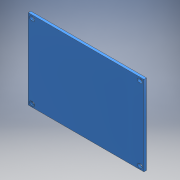
# Autodesk Inventor part: screen
Saved by Autodesk Inventor 2017 (Build 210142000, 142)
## iProperties
Part Number: screen
Material: Genérico
Document SubType Name: Modeling
Designer: Roberto
Density: 1 g/cm^3
Appearance: Valor por defecto
Author: Roberto
Autodesk Inventor part; units mm, degrees
ref_plane "YZ Plane" through (0, 0, 0) normal (1, 0, 0) x (0, 1, 0)
ref_plane "XZ Plane" through (0, 0, 0) normal (0, 1, 0) x (-1, 0, 0)
sketch "Boceto6" plane through (0, 0, 0) normal (0, 1, 0) x (-1, 0, 0)
  line L0 (0, 0) -> (8.94, 0)
  line L1 (8.94, 0) -> (8.94, -6.196)
  line L2 (8.94, -6.196) -> (0, -6.196)
  line L3 (0, -6.196) -> (0, 0)
  arc A0 (0.25, -0.1) -> (0.25, -0.4) centre (0.25, -0.25) ccw
  arc A1 (0.35, -0.4) -> (0.35, -0.1) centre (0.35, -0.25) ccw
  line L4 (0.25, -0.4) -> (0.35, -0.4)
  line L5 (0.25, -0.1) -> (0.35, -0.1)
  arc A2 (8.59, -0.1) -> (8.59, -0.4) centre (8.59, -0.25) ccw
  arc A3 (8.69, -0.4) -> (8.69, -0.1) centre (8.69, -0.25) ccw
  line L6 (8.59, -0.4) -> (8.69, -0.4)
  line L7 (8.59, -0.1) -> (8.69, -0.1)
  arc A4 (0.25, -5.796) -> (0.25, -6.096) centre (0.25, -5.946) ccw
  arc A5 (0.35, -6.096) -> (0.35, -5.796) centre (0.35, -5.946) ccw
  line L8 (0.25, -6.096) -> (0.35, -6.096)
  line L9 (0.25, -5.796) -> (0.35, -5.796)
  arc A6 (8.59, -5.796) -> (8.59, -6.096) centre (8.59, -5.946) ccw
  arc A7 (8.69, -6.096) -> (8.69, -5.796) centre (8.69, -5.946) ccw
  line L10 (8.59, -6.096) -> (8.69, -6.096)
  line L11 (8.59, -5.796) -> (8.69, -5.796)
  constraints: 24 end point, 16 point on circle, 8 centre point
extrude "Extrusión4" add sketch "Boceto6" along normal blind 0.6
sketch "Boceto7" plane through (0, 0.6, 0) normal (0, 1, 0) x (1, 0, 0)
  line L0 (-8.59, 5.796) -> (-8.69, 5.796) projected
  arc A0 (-8.69, 6.096) -> (-8.69, 5.796) centre (-8.69, 5.946) ccw projected
  line L1 (-8.69, 6.096) -> (-8.59, 6.096) projected
  arc A1 (-8.59, 5.796) -> (-8.59, 6.096) centre (-8.59, 5.946) ccw projected
  line L2 (-0.25, 5.796) -> (-0.35, 5.796) projected
  arc A2 (-0.35, 6.096) -> (-0.35, 5.796) centre (-0.35, 5.946) ccw projected
  line L3 (-0.35, 6.096) -> (-0.25, 6.096) projected
  arc A3 (-0.25, 5.796) -> (-0.25, 6.096) centre (-0.25, 5.946) ccw projected
  line L4 (-8.59, 0.1) -> (-8.69, 0.1) projected
  arc A4 (-8.69, 0.4) -> (-8.69, 0.1) centre (-8.69, 0.25) ccw projected
  line L5 (-8.69, 0.4) -> (-8.59, 0.4) projected
  arc A5 (-8.59, 0.1) -> (-8.59, 0.4) centre (-8.59, 0.25) ccw projected
  line L6 (-0.25, 0.1) -> (-0.35, 0.1) projected
  arc A6 (-0.35, 0.4) -> (-0.35, 0.1) centre (-0.35, 0.25) ccw projected
  line L7 (-0.35, 0.4) -> (-0.25, 0.4) projected
  arc A7 (-0.25, 0.1) -> (-0.25, 0.4) centre (-0.25, 0.25) ccw projected
  line L8 (-8.94, 0) -> (0, 0) projected
  line L9 (0, 0) -> (0, 6.196) projected
  line L10 (0, 6.196) -> (-8.94, 6.196) projected
  line L11 (-8.94, 6.196) -> (-8.94, 0) projected
  line L12 (-8.94, 6.196) -> (0, 6.196) projected
  line L13 (0, 0) -> (0, 6.196) projected
  line L14 (-0.8, 5.546) -> (-0.8, 0.65)
  line L15 (-0.8, 0.65) -> (-8.14, 0.65)
  line L16 (-8.14, 0.65) -> (-8.14, 5.546)
  line L17 (-8.14, 5.546) -> (-0.8, 5.546)
  constraints: 8 end point
extrude "Extrusión5" cut sketch "Boceto7" against normal blind 0.4
ref_plane "Plano de trabajo2" through (0, 2.3, 0) normal (0, 1, 0) x (1, 0, 0)
sketch "Boceto9" plane through (0, 2.3, 0) normal (0, 1, 0) x (1, 0, 0)
  line L0 (-8.4305, 5.546) -> (-0.2383, 5.546) construction
  line L1 (-0.2383, 5.546) -> (-0.2383, 0.5947) construction
  line L2 (-0.2383, 0.5947) -> (-8.4305, 0.5947) construction
  line L3 (-8.4305, 0.5947) -> (-8.4305, 5.546) construction
  line L4 (-0.8, 5.546) -> (-8.14, 5.546) projected
  line L5 (-8.14, 5.546) -> (-8.14, 0.65) projected
  line L6 (-8.14, 0.65) -> (-0.8, 0.65) projected
  line L7 (-0.8, 0.65) -> (-0.8, 5.546) projected
  point P0 (0, 0)
  constraints: 2 other
decal "Calcomanía1"
